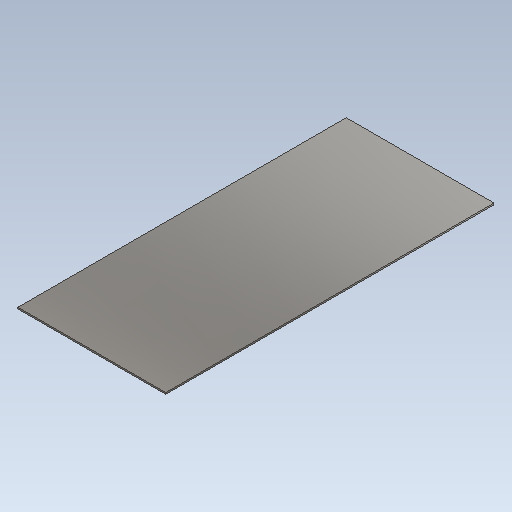
# Autodesk Inventor part: ADREF-000038
Saved by Autodesk Inventor 2020 (Build 240168000, 168)
## iProperties
Created: 2018-09-07
Part Number: ADREF-000038
Material: Steel, Mild
Description: Pump Set Mounting Plate
Document SubType Name: Modeling
Designer: alid
Stock Number: NA
Density: 7.85 g/cm^3
Appearance: Semi-Polished
Mass: 16249.5 g
Surface Area: 9133.4 cm^2
Volume: 2070 cm^3
Author: alid
Revision Number: A
Autodesk Inventor part; units mm, degrees
ref_plane "YZ Plane" through (0, 0, 0) normal (1, 0, 0) x (0, 1, 0)
ref_plane "XZ Plane" through (0, 0, 0) normal (0, 1, 0) x (-1, 0, 0)
ref_plane "XY Plane" through (0, 0, 0) normal (0, 0, 1) x (1, 0, 0)
sketch "Sketch1" plane through (0, 0, 0) normal (0, 0, 1) x (1, 0, 0)
  line L0 (-218.7206, -99.5962) -> (231.2794, -99.5962)
  line L1 (231.2794, -99.5962) -> (231.2794, 900.4038)
  line L2 (231.2794, 900.4038) -> (-218.7206, 900.4038)
  line L3 (-218.7206, 900.4038) -> (-218.7206, -99.5962)
  point P0 (0, 0)
  dimension "d0" = 450
  dimension "d1" = 1000
  constraints: 8 end point, 2 parallel, 1 horizontal, 1 perpendicular
  measures "d0" distance of L2.end L1.end
  measures "d1" distance of L1.end L0.end
extrude "Extrusion1" add sketch "Sketch1" along normal blind 4.6
body "Solid1"
